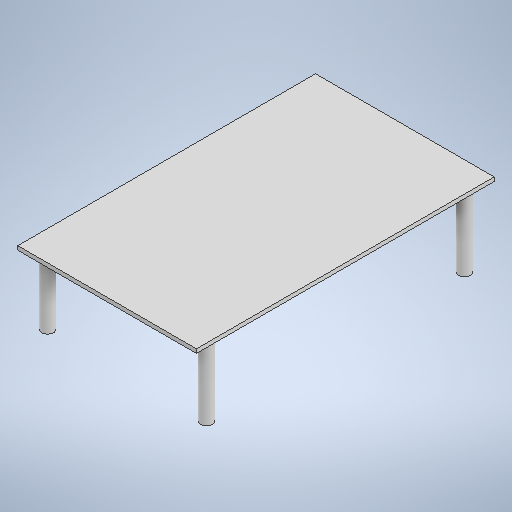
# Autodesk Inventor part: Support intérieur châssis
Saved by Autodesk Inventor 2026.2 (Build 302298010, 298A)
## iProperties
Created: 2026-04-13
Part Number: Support intérieur châssis
Material: Générique
Document SubType Name: Modeling
Designer: Genon
Density: 1 g/cm^3
Appearance: Par défaut
Author: Genon
Autodesk Inventor part; units mm, degrees
ref_plane "YZ Plane" through (0, 0, 0) normal (1, 0, 0) x (0, 1, 0)
ref_plane "XZ Plane" through (0, 0, 0) normal (0, 1, 0) x (-1, 0, 0)
ref_plane "XY Plane" through (0, 0, 0) normal (0, 0, 1) x (1, 0, 0)
sketch "Esquisse1" plane through (0, 0, 0) normal (0, 1, 0) x (-1, 0, 0)
  line L0 (0, 0) -> (0, 65)
  line L1 (0, 0) -> (0, -65)
  line L2 (0, 65) -> (40, 65)
  line L3 (-40, -65) -> (40, -65)
  circle A0 centre (40, 65) radius 3
  circle A1 centre (40, -65) radius 3
  circle A2 centre (-40, -65) radius 3
  line L4 (0, 65) -> (-40, 65)
  circle A3 centre (-40, 65) radius 3
  dimension "d0" = 65
  dimension "d1" = 65
  dimension "d2" = 40
  dimension "d4" = 80
  dimension "d5" = 6
  dimension "d7" = 6
  dimension "d9" = 6
  dimension "d11" = 40
  dimension "d12" = 6
  constraints: 10 end point, 4 centre point, 4 coincident, 2 horizontal, 2 vertical
  measures "d0" distance of L0.start L0.end
  measures "d1" distance of L0.start L1.end
  measures "d2" distance of L0.end L2.end
  measures "d4" distance of L3.start L3.end
  measures "d5" diameter of A0
  measures "d7" diameter of A1
  measures "d9" diameter of A2
  measures "d11" distance of L0.end L4.end
  measures "d12" diameter of A3
extrude "Extrusion1" add sketch "Esquisse1" along normal blind 37
sketch "Esquisse2" plane through (-40, 37, 65) normal (0, 1, 0) x (1, 0, 0)
  line L0 (0, 0) -> (80, 0)
  line L1 (80, 0) -> (80, 130)
  line L2 (80, 130) -> (0, 130)
  line L3 (0, 130) -> (0, 0)
  line L4 (0, 0) -> (0, -10)
  line L5 (0, -10) -> (85, -10)
  line L6 (85, -10) -> (85, 140)
  line L7 (85, 140) -> (-5, 140)
  line L8 (-5, 140) -> (-5, -10)
  line L9 (-5, -10) -> (0, -10)
  point P0 (40, 65)
  dimension "d16" = 80
  dimension "d17" = 130
  dimension "d18" = 10
  dimension "d19" = 85
  dimension "d20" = 150
  dimension "d21" = 90
  constraints: 20 end point, 6 perpendicular, 2 parallel, 1 horizontal, 1 point on line, 1 vertical
  measures "d16" distance of L2.end L1.end
  measures "d17" distance of L1.end L0.end
  measures "d18" distance of L0.start L4.end
  measures "d19" distance of L4.end L5.end
  measures "d20" distance of L5.end L6.end
  measures "d21" distance of L6.end L7.end
extrude "Extrusion2" add sketch "Esquisse2" along normal blind 2 contours L3 L2 L1 L0 | L9 L8 L7 L6 L5
sketch "Esquisse3" plane through (40, 0, 65) normal (0, -1, 0) x (1, 0, 0)
  circle A0 centre (0, -130) radius 3 projected
  circle A1 centre (-80, 0) radius 3 projected
  circle A2 centre (-80, -130) radius 3 projected
  point P0 (-40, -65)
  point P1 (0, 0)
  constraints: 3 coincident
hole "Perçage1" at (40, 0, 65) at (40, 0, -65) at (-40, 0, 65) at (-40, 0, -65) direction (0, 1, 0) diameter 2.459 depth 30 thread size "M3x0.5" class "6H" standard "ISO Metric profile"
